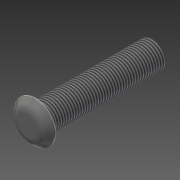
# Autodesk Inventor part: Rdzeń_wentyla
Saved by Autodesk Inventor 2015 (Build 190159000, 159)
## iProperties
Created: 2015-12-01
Part Number: Rdzeń_wentyla
Material: Aluminium AW-7020
Document SubType Name: Modeling
Designer: graaapsik
Density: 2.78 g/cm^3
Appearance: Aluminium AW-7020
Mass: 3.9105 g
Surface Area: 15.02 cm^2
Volume: 1.40665 cm^3
Author: graaapsik
Autodesk Inventor part; units mm, degrees
ref_plane "YZ Plane" through (0, 0, 0) normal (1, 0, 0) x (0, 1, 0)
ref_plane "XZ Plane" through (0, 0, 0) normal (0, 1, 0) x (-1, 0, 0)
ref_plane "XY Plane" through (0, 0, 0) normal (0, 0, 1) x (1, 0, 0)
sketch "Szkic1" plane through (0, 0, 0) normal (0, 1, 0) x (-1, 0, 0)
  circle A0 centre (0, 0) radius 4
  dimension "d0" = 8
  constraints: 1 centre point, 1 coincident
  measures "d0" diameter of A0
extrude "Wyciągnięcie proste1" add sketch "Szkic1" along normal mid plane 35
sketch "Szkic3" plane through (0, 0, 0) normal (1, 0, 0) x (0, 1, 0)
  line L0 (-17.5, 4) -> (-17.5, -4) construction
  line L1 (-17.5, 0) -> (-17.5, 5.7452)
  line L2 (-18.363, 6.0891) -> (-19.3779, 5.0178)
  line L3 (-20.2, 2.9546) -> (-20.2, 0)
  line L4 (-20.2, 0) -> (-17.5, 0)
  arc A0 (-19.3779, 5.0178) -> (-20.2, 2.9546) centre (-17.2, 2.9546) ccw
  arc A1 (-17.5, 5.7452) -> (-18.363, 6.0891) centre (-18, 5.7452) ccw
  line L5 (-17.5, 0) -> (-13.3351, 0) construction
  point P0 (0, 0)
  point P1 (-17.5, 7)
  point P2 (-20.2, 4.15)
  dimension "d3" = 7
  dimension "d4" = 2.7
  dimension "d5" = 4.15
  dimension "d6" = 3
  dimension "d7" = 0.5
  constraints: 10 end point, 5 point on line, 4 point on circle, 4 tangent, 2 centre point, 1 collinear, 1 midpoint, 1 parallel, 1 perpendicular
  measures "d3" distance of L1.start point (-17.5, 7)
  measures "d4" distance of L3.end L1.start
  measures "d5" distance of point (-20.2, 4.15) L3.end
  measures "d6" radius of A0
  measures "d7" radius of A1
revolve "Podstawa" add sketch "Szkic3" angle 360 about axis through (0, -17.5, 0) along (0, 1, 0)
thread "Gwint1" size "M8x0.8" class "6g" standard "ISO Metric profile" full length
sketch "Szkic4" plane through (0, 17.5, 0) normal (0, 1, 0) x (1, 0, 0)
  circle A0 centre (0, 0) radius 4 projected
  constraints: 1 coincident
hole "Otwór1" at (0, 17.5, 0) direction (0, -1, 0) diameter 7 depth 15 tip angle 118
